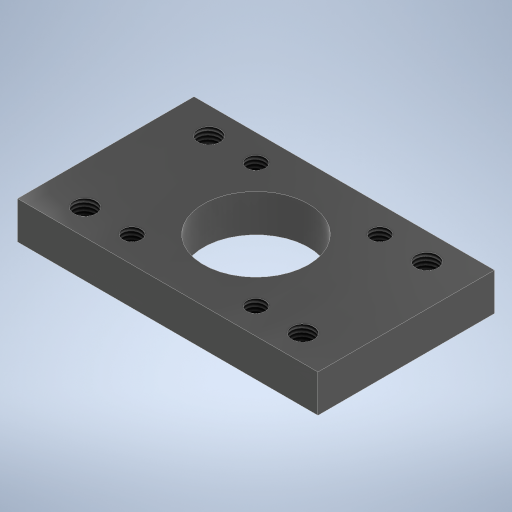
# Autodesk Inventor part: 2309HCMUTE-CDT23-GA_SC32
Saved by Autodesk Inventor 2023 (Build 270158000, 158)
## iProperties
Created: 2023-11-16
Part Number: 2309HCMUTE-CDT23-GA_SC32
Material: PPS Plastic
Document SubType Name: Sheet Metal
Designer: havie
Density: 1.637 g/cm^3
Sheet Metal Rule: Default_mm
Appearance: Dark Gray
Author: havie
Autodesk Inventor part; units mm, degrees
ref_plane "YZ Plane" through (0, 0, 0) normal (1, 0, 0) x (0, 1, 0)
ref_plane "XZ Plane" through (0, 0, 0) normal (0, 1, 0) x (-1, 0, 0)
ref_plane "XY Plane" through (0, 0, 0) normal (0, 0, 1) x (1, 0, 0)
sketch "Sketch1" plane through (0, 0, 0) normal (0, 1, 0) x (-1, 0, 0)
  line L0 (40, 23.5) -> (-40, 23.5)
  line L1 (-40, 23.5) -> (-40, -23.5)
  line L2 (-40, -23.5) -> (40, -23.5)
  line L3 (40, -23.5) -> (40, 23.5)
  line L4 (40, 23.5) -> (-40, -23.5) construction
  line L5 (-40, 23.5) -> (40, -23.5) construction
  point P0 (0, 0)
  dimension "d0" = 80
  dimension "d1" = 47
  measures "d0" distance of L1.end L2.end
  measures "d1" distance of L0.end L1.end
extrude "Plate1" add sketch "Sketch1" along normal mid plane 10
sketch "Sketch2" plane through (0, 5, 0) normal (0, 1, 0) x (1, 0, 0)
  point P0 (0, 0)
  point P1 (-29, -16.5)
  point P2 (-29, 16.5)
  point P3 (29, 16.5)
  point P4 (29, -16.5)
  dimension "d3" = 58
  dimension "d4" = 33
  dimension "d5" = 16.5
  dimension "d6" = 29
  constraints: 2 horizontal alignment, 2 vertical alignment
  measures "d3" distance of point (29, -16.5) point (-29, -16.5)
  measures "d4" distance of point (29, -16.5) point (29, 16.5)
  measures "d5" vertical distance of point (-29, -16.5) point (0, 0)
  measures "d6" horizontal distance of point (0, 0) point (-29, -16.5)
hole "Hole1" at (-29, 5, 16.5) at (-29, 5, -16.5) at (29, 5, -16.5) at (29, 5, 16.5) direction (0, -1, 0) diameter 5.9175 depth 19.1 tip angle 118 thread size "M7x1" class "6H" standard "ISO Metric profile"
sketch "Sketch3" plane through (0, 5, 0) normal (0, 1, 0) x (1, 0, 0)
  point P0 (0, 0)
  point P1 (-16.5, -16.5)
  point P2 (-16.5, 16.5)
  point P3 (16.5, 16.5)
  point P4 (16.5, -16.5)
  dimension "d14" = 33
  dimension "d15" = 33
  dimension "d16" = 16.5
  dimension "d17" = 16.5
  constraints: 2 horizontal alignment, 2 vertical alignment
  measures "d14" distance of point (16.5, 16.5) point (16.5, -16.5)
  measures "d15" distance of point (-16.5, 16.5) point (16.5, 16.5)
  measures "d16" horizontal distance of point (0, 0) point (16.5, 16.5)
  measures "d17" horizontal distance of point (0, 0) point (16.5, 16.5)
hole "Hole2" at (-16.5, 5, 16.5) at (-16.5, 5, -16.5) at (16.5, 5, -16.5) at (16.5, 5, 16.5) direction (0, -1, 0) diameter 4.917 depth 17.1 tip angle 118 thread size "M6x1" class "6H" standard "ISO Metric profile"
sketch "Sketch4" plane through (0, 5, 0) normal (0, 1, 0) x (1, 0, 0)
  circle A0 centre (0, 0) radius 14
  dimension "d25" = 28
  constraints: 1 centre point, 1 coincident
  measures "d25" diameter of A0
extrude "Cut1" cut sketch "Sketch4" against normal blind 10
equation "\"d26\" = Thickness"
equation "\"d2\" = Thickness"
equation "\"BendReliefDepth\" = 0.5 * Thickness"
equation "\"Thickness\" = 10"
body "Solid1"
